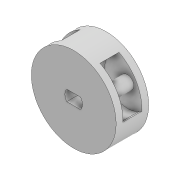
# Autodesk Inventor part: Pump_Rotatio_new.
Saved by Autodesk Inventor 2022.5 (Build 265521000, 521)
## iProperties
Created: 2022-11-30
Part Number: Pump_Rotatio_new.
Material: Generisch
Document SubType Name: Modeling
Designer: diederichbenedict
Density: 1 g/cm^3
Appearance: Vorgabe
Author: diederichbenedict
Autodesk Inventor part; units mm, degrees
ref_plane "YZ Plane" through (0, 0, 0) normal (1, 0, 0) x (0, 1, 0)
ref_plane "XZ Plane" through (0, 0, 0) normal (0, 1, 0) x (-1, 0, 0)
ref_plane "XY Plane" through (0, 0, 0) normal (0, 0, 1) x (1, 0, 0)
sketch "Skizze3" plane through (0, 0, 0) normal (0, 0, 1) x (1, 0, 0)
  circle A0 centre (82.735856, -97.364718) radius 1.5
  circle A1 centre (87.344144, -89.642424) radius 2.777622
  circle A2 centre (0, 0) radius 12.5
  line L0 (0, -9.5) -> (-8.227241, 4.75)
  line L1 (-8.227241, 4.75) -> (8.227241, 4.75)
  line L2 (8.227241, 4.75) -> (0, -9.5)
  circle A3 centre (0, -9.5) radius 1.9
  circle A4 centre (8.227241, 4.75) radius 1.9
  circle A5 centre (-8.227241, 4.75) radius 1.9
  circle A6 centre (0, 0) radius 2.6
  line L3 (-2.04939, -1.6) -> (2.04939, -1.6)
  line L4 (-2.04939, 1.6) -> (2.04939, 1.6)
  circle A7 centre (8.227241, 4.75) radius 2 construction
  dimension "d10" = 25
  dimension "d11" = 9.5
  dimension "d12" = 3.8
  dimension "d13" = 3.8
  dimension "d14" = 3.8
  dimension "d15" = 5.2
  dimension "d16" = 1.6
  dimension "d17" = 1.6
  constraints: 10 end point, 6 coincident, 5 centre point, 4 point on circle, 1 horizontal, 7 other
  measures "d10" diameter of A2
  measures "d11" distance of L0.start point (0, 0)
  measures "d12" diameter of A3
  measures "d13" diameter of A4
  measures "d14" diameter of A5
  measures "d15" diameter of A6
  measures "d16" distance from line of point (0, 0) L3
  measures "d17" distance from line of L4 A2.centre
sketch "Skizze3 outline for Extrusion3" plane through (0, 0, 0) normal (0, 0, 1) x (1, 0, 0)
  circle A0 centre (0, 0) radius 12.5
  circle A1 centre (0, -9.5) radius 1.9
  arc A2 (2.04939, 1.6) -> (2.04939, -1.6) centre (0, 0) cw
  line L0 (-2.04939, 1.6) -> (2.04939, 1.6)
  arc A3 (-2.04939, -1.6) -> (-2.04939, 1.6) centre (0, 0) cw
  line L1 (2.04939, -1.6) -> (-2.04939, -1.6)
  circle A4 centre (-8.227241, 4.75) radius 1.9
  circle A5 centre (8.227241, 4.75) radius 1.9
extrude "Extrusion3" add sketch "Skizze3 outline for Extrusion3" along normal blind 2
sketch "Skizze4" plane through (0, 0, 0) normal (0, 0, -1) x (-1, 0, 0)
  circle A0 centre (0, 0) radius 12.5
  circle A1 centre (8.227241, 4.75) radius 1.9
  circle A2 centre (0, -9.5) radius 1.9
  arc A3 (-2.04939, 1.6) -> (-2.04939, -1.6) centre (0, 0) ccw
  line L0 (2.04939, 1.6) -> (-2.04939, 1.6)
  arc A4 (2.04939, -1.6) -> (2.04939, 1.6) centre (0, 0) ccw
  line L1 (-2.04939, -1.6) -> (2.04939, -1.6)
  circle A5 centre (-8.227241, 4.75) radius 1.9
  circle A6 centre (0, -9.5) radius 6.75
  circle A7 centre (-8.227241, 4.75) radius 6.75
  circle A8 centre (8.227241, 4.75) radius 6.75
  line L2 (-6.75, -16.25) -> (6.7082, -16.25)
  line L3 (6.7082, -16.25) -> (6.7082, -8.749965)
  line L4 (6.7082, -8.749965) -> (-6.75, -8.749965)
  line L5 (-6.75, -8.749965) -> (-6.75, -16.25)
  line L6 (-6.75, -16.25) -> (6.7082, -8.749965) construction
  line L7 (6.7082, -16.25) -> (-6.75, -8.749965) construction
  line L8 (5.75657, -4.470671) -> (17.447913, 2.279329)
  line L9 (17.447913, 2.279329) -> (10.697913, 13.970671)
  line L10 (10.697913, 13.970671) -> (-0.99343, 7.220671)
  line L11 (-0.99343, 7.220671) -> (5.75657, -4.470671)
  line L12 (5.75657, -4.470671) -> (10.697913, 13.970671) construction
  line L13 (17.447913, 2.279329) -> (-0.99343, 7.220671) construction
  line L14 (0, 0) -> (8.227241, 4.75)
  line L15 (8.227241, 4.75) -> (0, 0)
  line L16 (0, 0) -> (-8.263885, 4.771156)
  line L17 (-5.75657, -4.470671) -> (0.99343, 7.220671)
  line L18 (0.99343, 7.220671) -> (-10.7712, 14.012984)
  line L19 (-10.7712, 14.012984) -> (-17.5212, 2.321641)
  line L20 (-17.5212, 2.321641) -> (-5.75657, -4.470671)
  line L21 (-5.75657, -4.470671) -> (-10.7712, 14.012984) construction
  line L22 (0.99343, 7.220671) -> (-17.5212, 2.321641) construction
  point P0 (5.826917, 11.058799)
  point P1 (12.490659, -0.483141)
  point P2 (-5.826917, 11.058799)
  point P3 (-12.490659, -0.483141)
  point P4 (-6.663742, -10.575658)
  point P5 (6.663742, -10.575658)
  point P6 (-0.0209, -12.499983)
  point P7 (-11.602241, -1.095671)
  point P8 (-12.486291, -0.585265)
  point P9 (-6.75, -10.520813)
  point P10 (-6.75, -9.5)
  point P11 (6.7082, -10.547514)
  point P12 (12.486291, -0.585265)
  point P13 (11.602241, -1.095671)
  point P14 (4.852241, 10.595671)
  point P15 (5.736291, 11.106078)
  point P16 (-5.736291, 11.106078)
  point P17 (-4.852241, 10.595671)
  dimension "d20" = 13.5
  dimension "d21" = 13.5
  dimension "d22" = 13.5
  constraints: 42 end point, 7 parallel, 6 midpoint, 5 tangent, 4 perpendicular, 3 coincident, 2 centre point, 2 horizontal, 1 collinear, 1 vertical, 5 other
  measures "d21" diameter of A7
  measures "d22" diameter of A8
sketch "Skizze4 outline for Extrusion4" plane through (0, 0, 0) normal (0, 0, -1) x (-1, 0, 0)
  line L0 (-11.602241, -1.095671) -> (-12.486291, -0.585265)
  arc A0 (-4.852241, 10.595671) -> (-11.602241, -1.095671) centre (-8.227241, 4.75) cw
  arc A1 (-12.486291, -0.585265) -> (-6.75, -10.520813) centre (0, 0) ccw
  line L1 (-5.736291, 11.106078) -> (-4.852241, 10.595671)
  line L2 (-6.75, -10.520813) -> (-6.75, -9.5)
  arc A2 (5.736291, 11.106078) -> (-5.736291, 11.106078) centre (0, 0) ccw
  arc A3 (-6.75, -9.5) -> (6.7082, -8.749965) centre (0, -9.5) cw
  line L3 (4.852241, 10.595671) -> (5.736291, 11.106078)
  line L4 (6.7082, -8.749965) -> (6.7082, -10.547514)
  arc A4 (11.602241, -1.095671) -> (4.852241, 10.595671) centre (8.227241, 4.75) cw
  arc A5 (6.7082, -10.547514) -> (12.486291, -0.585265) centre (0, 0) ccw
  line L5 (12.486291, -0.585265) -> (11.602241, -1.095671)
  arc A6 (-2.04939, -1.6) -> (-2.04939, 1.6) centre (0, 0) cw
  line L6 (2.04939, -1.6) -> (-2.04939, -1.6)
  arc A7 (2.04939, 1.6) -> (2.04939, -1.6) centre (0, 0) cw
  line L7 (-2.04939, 1.6) -> (2.04939, 1.6)
extrude "Extrusion4" add sketch "Skizze4 outline for Extrusion4" along normal blind 2.8
sketch "Skizze9" plane through (0, 0, 0) normal (0, 0, -1) x (-1, 0, 0)
  circle A0 centre (-8.227241, 4.75) radius 1.9
  circle A1 centre (8.227241, 4.75) radius 1.9
  circle A2 centre (0, -9.5) radius 1.9
  point P0 (0, 0)
sketch "Skizze9 outline for Extrusion7" plane through (0, 0, 0) normal (0, 0, -1) x (-1, 0, 0)
  circle A0 centre (0, -9.5) radius 1.9
  circle A1 centre (8.227241, 4.75) radius 1.9
  circle A2 centre (-8.227241, 4.75) radius 1.9
extrude "Extrusion7" add sketch "Skizze9 outline for Extrusion7" along normal blind 2.8 and the other way blind 2
mirror "Spiegeln1" about plane through (0, 0.976243, -2.8) normal (0, 0, -1) of "Extrusion3", "Extrusion4", "Extrusion7"
equation "\"d12\" = d13"
equation "\"d14\" = d13"
equation "\"d17\" = d16"
equation "\"d20\" = d21"
equation "\"d22\" = d21"
